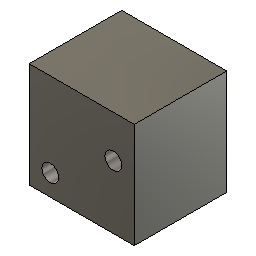
AltIMU Bracket v1 (Autodesk Fusion 360 design; units mm, degrees)
Autodesk Fusion 360 part; units mm, degrees
sketch "Sketch1" plane through (0, 0, 0) normal (0, 0, 1) x (1, 0, 0)
  line L0 (0, 0) -> (12.7, 0)
  line L1 (12.7, 0) -> (12.7, 12.7)
  line L2 (12.7, 12.7) -> (0, 12.7)
  line L3 (0, 12.7) -> (0, 0)
  circle A0 centre (2.54, 2.54) radius 1.016
  circle A1 centre (10.16, 7.62) radius 1.016
  dimension "d1" = 12.7
  dimension "d2" = 12.7
  dimension "d3" = 2.032
  dimension "d4" = 2.54
  dimension "d5" = 2.54
  dimension "d6" = 2.032
  dimension "d7" = 2.54
  dimension "d8" = 5.08
  constraint horizontal L0
  constraint vertical L1
  constraint horizontal L2
  constraint vertical L3
  constraint coincident L0.start L3.end
  measures "d1" distance of L0.start L0.end
  measures "d2" distance of L0.start L2.end
  measures "d3" diameter of A0
  measures "d4" distance of L0 A0.centre
  measures "d5" distance of L3 A0.centre
  measures "d6" diameter of A1
  measures "d7" distance of L1 A1.centre
  measures "d8" distance of L2 A1.centre
extrude "Extrude1" add sketch "Sketch1" along normal blind 11.176
